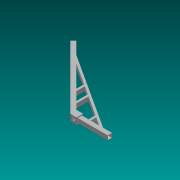
# Autodesk Inventor part: kepala baru
Saved by Autodesk Inventor 2014 SP2 (Build 180246200, 246)
## iProperties
Created: 2019-07-15
Part Number: kepala baru
Material: Steel, Mild
Document SubType Name: Modeling
Designer: USER PC
Density: 7.86 g/cm^3
Appearance: Steel
Author: USER PC
Autodesk Inventor part; units mm, degrees
ref_plane "YZ Plane" through (0, 0, 0) normal (1, 0, 0) x (0, 1, 0)
ref_plane "XZ Plane" through (0, 0, 0) normal (0, 1, 0) x (-1, 0, 0)
ref_plane "XY Plane" through (0, 0, 0) normal (0, 0, 1) x (1, 0, 0)
sketch "Sketch1" plane through (0, 0, 0) normal (0, 0, 1) x (1, 0, 0)
  line L0 (0, 0) -> (150, 0)
  line L1 (150, 0) -> (150, 150)
  line L2 (150, 150) -> (0, 150)
  line L3 (0, 150) -> (0, 0)
  line L4 (0, 0) -> (-1500, 1500)
  line L5 (-1500, 1500) -> (-1429.2893, 1570.7107)
  line L6 (-1429.2893, 1570.7107) -> (0, 141.4214)
  line L7 (0, 141.4214) -> (0, 0)
  line L8 (150, 100) -> (150, 0)
  line L9 (150, 0) -> (150, 125)
  line L10 (150, 125) -> (850, 125)
  line L11 (850, 125) -> (850, 25)
  line L12 (850, 25) -> (150, 25)
  line L13 (150, 25) -> (150, 125)
  dimension "d0" = 150
  dimension "d1" = 150
  dimension "d8" = 1500
  dimension "d9" = 100
  dimension "d12" = 125
  dimension "d13" = 700
  dimension "d14" = 100
  constraints: 28 end point, 5 perpendicular, 4 parallel, 1 collinear, 1 horizontal, 1 point on line
  measures "d0" distance of L2.end L1.end
  measures "d1" distance of L1.end L0.end
  measures "d8" horizontal distance of L0.start L4.end
  measures "d9" distance of L4.end L5.end
  measures "d12" distance of L0.end L9.end
  measures "d13" distance of L9.end L10.end
  measures "d14" distance of L10.end L11.end
extrude "Extrusion3" add sketch "Sketch1" along normal mid plane 150 contours L3 L2 L1 L0
sketch "Sketch3" plane through (0, 0, 0) normal (0, 0, 1) x (1, 0, 0)
  line L0 (0, 0) -> (-1500, 1500)
  line L1 (0, 0) -> (2121.3203, 0) construction
  line L2 (-1500, 1500) -> (-1429.2893, 1570.7107)
  line L3 (-1429.2893, 1570.7107) -> (0, 141.4214)
  line L4 (0, 0) -> (0, 141.4214)
  line L5 (150, 0) -> (150, 125)
  line L6 (150, 125) -> (850, 125)
  line L7 (850, 125) -> (850, 25)
  line L8 (850, 25) -> (150, 25)
  line L9 (150, 25) -> (150, 125)
  dimension "d17" = 135
  dimension "d18" = 1500
  dimension "d19" = 100
  dimension "d20" = 125
  dimension "d21" = 700
  dimension "d22" = 100
  constraints: 20 end point, 5 perpendicular, 3 parallel, 1 equal length, 1 horizontal, 1 point on line
  measures "d17" angle of L1 L0
  measures "d18" horizontal distance of L0.start L0.end
  measures "d19" distance of L0.end L2.end
  measures "d20" distance of L5.start L5.end
  measures "d21" distance of L5.end L6.end
  measures "d22" distance of L6.end L7.end
extrude "Extrusion4" add sketch "Sketch3" along normal mid plane 100
sketch "Sketch4" plane through (-1500, 1500, -50) normal (-0.7071, 0.7071, 0) x (-0.7071, -0.7071, 0)
  line L0 (-95, 95) -> (-5, 95)
  line L1 (-5, 95) -> (-5, 5)
  line L2 (-5, 5) -> (-95, 5)
  line L3 (-95, 5) -> (-95, 95)
  line L4 (-95, 95) -> (-5, 5) construction
  line L5 (-5, 95) -> (-95, 5) construction
  point P0 (0, 50)
  point P1 (-50, 50)
  dimension "d25" = 90
  dimension "d26" = 90
  constraints: 12 end point, 2 midpoint, 2 parallel, 1 horizontal, 1 perpendicular
  measures "d25" distance of L1.end L2.end
  measures "d26" distance of L0.end L1.end
extrude "Extrusion5" cut sketch "Sketch4" against normal blind 2122.5
sketch "Sketch5" plane through (0, 0, 0) normal (0, 0, 1) x (1, 0, 0)
  line L0 (0, 132.8216) -> (69.0672, 132.8216)
  line L1 (69.0672, 132.8216) -> (69.0672, 2.6564)
  line L2 (69.0672, 2.6564) -> (0, 2.6564)
  line L3 (0, 2.6564) -> (0, 132.8216)
  point P0 (0, 0)
  constraints: 8 end point, 2 parallel, 1 horizontal, 1 perpendicular
extrude "Extrusion6" add sketch "Sketch5" along normal mid plane 100.5
sketch "Sketch6" plane through (0, 0, 0) normal (0, 0, 1) x (1, 0, 0)
  point P0 (0, 0)
sketch "Sketch7" plane through (0, 150, 75) normal (0, 1, 0) x (1, 0, 0)
  circle A0 centre (75, 75) radius 30
  point P0 (0, 75)
  dimension "d31" = 60
  constraints: 1 centre point
  measures "d31" diameter of A0
extrude "Extrusion7" cut sketch "Sketch7" against normal blind 340
sketch "Sketch8" plane through (850, 25, 50) normal (1, 0, 0) x (0, 0, -1)
  line L0 (5, 95) -> (95, 95)
  line L1 (95, 95) -> (95, 5)
  line L2 (95, 5) -> (5, 5)
  line L3 (5, 5) -> (5, 95)
  line L4 (5, 95) -> (95, 5) construction
  line L5 (95, 95) -> (5, 5) construction
  point P0 (50, -25)
  point P1 (50, 50)
  dimension "d34" = 90
  dimension "d35" = 90
  constraints: 12 end point, 2 midpoint, 2 parallel, 1 horizontal, 1 perpendicular
  measures "d34" distance of L1.end L2.end
  measures "d35" distance of L0.end L1.end
extrude "Extrusion8" cut sketch "Sketch8" against normal blind 700
sketch "Sketch9" plane through (0, 0, 0) normal (0, 0, 1) x (1, 0, 0)
  point P0 (0, 0)
sketch "Sketch10" plane through (0, 0, 0) normal (0, 0, 1) x (1, 0, 0)
  line L0 (150, 125) -> (550, 125)
  line L1 (550, 125) -> (-971.9923, 1113.3934)
  line L2 (550, 125) -> (2376.4621, 125) construction
  line L3 (550, 125) -> (641.8039, 125)
  line L4 (641.8039, 125) -> (-1142.0421, 1283.4431)
  line L5 (-971.9923, 1113.3934) -> (-1142.0421, 1283.4431)
  line L6 (-971.9923, 1113.3934) -> (-731.5056, 1113.3934) construction
  line L7 (150, 125) -> (300, 125)
  point P0 (0, 0)
  dimension "d41" = 147
  dimension "d42" = 50
  dimension "d43" = 400
  dimension "d44" = 135
  dimension "d45" = 150
  constraints: 16 end point, 3 horizontal, 2 point on line, 1 equal length, 1 parallel
  measures "d41" angle of L2 L1
  measures "d42" distance between parallel lines of L4 L1
  measures "d43" distance of L0.start L0.end
  measures "d44" angle of L6 L5
  measures "d45" distance of L0.start L7.end
extrude "Extrusion9" add sketch "Sketch10" along normal mid plane 100
sketch "Sketch11" plane through (0, 0, 50) normal (0, 0, 1) x (1, 0, 0)
  line L0 (0, 141.4214) -> (-971.9344, 1113.3558) projected
  line L1 (-971.9344, 1113.3558) -> (550, 125) projected
  line L2 (550, 125) -> (150, 125) projected
  line L3 (150, 125) -> (300, 125)
  line L4 (300, 125) -> (300, 287.3519)
  line L5 (300, 125) -> (350, 125)
  line L6 (350, 125) -> (350, 254.8815)
  line L7 (300, 287.3519) -> (350, 254.8815)
  line L8 (305, 130) -> (305, 278.143)
  line L9 (0, 141.4214) -> (-212.132, 353.5534)
  line L10 (-212.132, 353.5534) -> (-247.4874, 388.9087)
  line L11 (-93.5014, 542.8947) -> (-50.6311, 515.0544)
  line L12 (0, 141.4214) -> (-459.6194, 601.0408)
  line L13 (-459.6194, 601.0408) -> (-494.9747, 636.3961)
  line L14 (-212.132, 353.5534) -> (-212.132, 619.9343)
  line L15 (-162.132, 303.5534) -> (-162.132, 587.464)
  line L16 (-212.132, 353.5534) -> (-175.196, 316.6173)
  line L17 (-212.132, 619.9343) -> (-162.132, 587.464)
  line L18 (-459.6194, 601.0408) -> (-459.6194, 780.6545)
  line L19 (-409.6194, 748.1841) -> (-409.6194, 551.0408)
  line L20 (-409.6194, 551.0408) -> (-459.6194, 601.0408)
  line L21 (-409.6194, 551.0408) -> (-459.6194, 601.0408)
  line L22 (-459.6194, 601.0408) -> (-409.6194, 551.0408)
  line L23 (-459.6194, 780.6545) -> (-409.6194, 748.1841)
  dimension "d48" = 150
  dimension "d49" = 50
  dimension "d51" = 300
  dimension "d52" = 50
  dimension "d54" = 650
  dimension "d55" = 50
  dimension "d71" = 50
  dimension "d72" = 50
  constraints: 42 end point, 8 point on line, 4 parallel, 3 collinear, 2 perpendicular, 1 midpoint, 12 other
  measures "d48" distance of L2.end L3.end
  measures "d49" distance of L3.end L5.end
  measures "d51" distance of L0.start L9.end
  measures "d52" distance of L9.end L10.end
  measures "d54" distance of L0.start L12.end
  measures "d55" distance of L12.end L13.end
  measures "d71" distance between parallel lines of L15 L14
  measures "d72" distance between parallel lines of L19 L18
sketch "Sketch13" plane through (0, 0, 50) normal (0, 0, 1) x (1, 0, 0)
  line L0 (-314.5783, 746.0819) -> (-298.0455, 762.6147) projected
  line L1 (-333.4008, 797.97) -> (-298.0455, 762.6147) projected
  line L2 (-357.4486, 773.9222) -> (-333.4008, 797.97) projected
  line L3 (-971.9344, 1113.3558) -> (550, 125) projected
  line L4 (-314.5783, 746.0819) -> (-357.4486, 773.9222)
  line L5 (-333.4008, 797.97) -> (-298.0455, 762.6147)
  line L6 (-298.0455, 762.6147) -> (-314.5783, 746.0819)
  line L7 (-333.4008, 797.97) -> (-357.4486, 773.9222)
  point P0 (-393.5938, 737.777)
  constraints: 8 end point, 1 collinear, 1 parallel, 1 perpendicular, 1 point on line
extrude "Extrusion11" cut sketch "Sketch13" against normal blind 228.5
sketch "Sketch16" plane through (0, 0, 0) normal (0, 0, 1) x (1, 0, 0)
  point P0 (0, 0)
extrude "Extrusion13" add sketch "Sketch11" against normal blind 100 contours L1 L6 L2 L4 | L0 L14 L1 L15 | L19 L0 L18 L1
body "Solid1"
